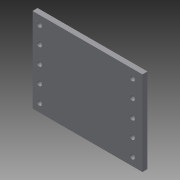
# Autodesk Inventor part: 知能ロボコン敷板
Saved by Autodesk Inventor 2013 (Build 170138000, 138)
## iProperties
Created: 2014-05-21
Part Number: 知能ロボコン敷板
Material: 一般
Document SubType Name: Modeling
Designer: horumo136
Density: 1 g/cm^3
Author: horumo136
Autodesk Inventor part; units mm, degrees
ref_plane "YZ Plane" through (0, 0, 0) normal (1, 0, 0) x (0, 1, 0)
ref_plane "XZ Plane" through (0, 0, 0) normal (0, 1, 0) x (-1, 0, 0)
ref_plane "XY Plane" through (0, 0, 0) normal (0, 0, 1) x (1, 0, 0)
sketch "スケッチ1" plane through (0, 0, 0) normal (0, 1, 0) x (-1, 0, 0)
  line L0 (0, 0) -> (-65, 0)
  line L1 (-65, 0) -> (-65, 50)
  line L2 (-65, 50) -> (0, 50)
  line L3 (0, 50) -> (0, 0)
  dimension "d0" = 65
  dimension "d1" = 50
  constraints: 8 end point, 2 parallel, 1 horizontal, 1 perpendicular
  measures "d0" distance of L1.end L2.end
  measures "d1" distance of L0.end L1.end
extrude "押し出し1" add sketch "スケッチ1" along normal blind 3
sketch "スケッチ2" plane through (0, 3, 0) normal (0, 1, 0) x (1, 0, 0)
  line L0 (65, 0) -> (0, 0) projected
  line L1 (0, 0) -> (0, -50) projected
  line L2 (0, -50) -> (65, -50) projected
  line L3 (65, -50) -> (65, 0) projected
  line L4 (59, 0) -> (59, -50)
  line L5 (4, 0) -> (4, -50)
  line L6 (0, -25) -> (65, -25)
  point P0 (59, -25)
  point P1 (59, -15)
  point P2 (59, -5)
  point P3 (59, -35)
  point P4 (59, -45)
  point P5 (4, -25)
  point P6 (4, -15)
  point P7 (4, -5)
  point P8 (4, -35)
  point P9 (4, -45)
  point P10 (4, -25)
  dimension "d4" = 6
  dimension "d5" = 55
  dimension "d6" = 10
  dimension "d7" = 10
  constraints: 12 point on line, 6 end point, 4 midpoint, 2 symmetric about line, 1 coincident, 1 parallel, 1 perpendicular
  measures "d4" distance between parallel lines of L3 L4
  measures "d5" distance between parallel lines of L4 L5
  measures "d6" distance of point (59, -25) point (59, -15)
  measures "d7" distance of point (59, -5) point (59, -15)
hole "穴1" at (59, 3, 25) at (59, 3, 15) at (59, 3, 5) at (59, 3, 45) at (59, 3, 35) at (4, 3, 25) at (4, 3, 15) at (4, 3, 5) at (4, 3, 35) at (4, 3, 45) direction (0, -1, 0) diameter 3 depth 8 tip angle 118
